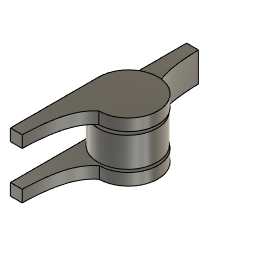
My_hinge (Autodesk Fusion 360 design; units mm, degrees)
Autodesk Fusion 360 part; units mm, degrees
sketch "Sketch1" plane through (0, 0, 0) normal (0, 0, 1) x (1, 0, 0)
  line L0 (-3, 15) -> (-5, 15)
  line L1 (-5, 15) -> (-5, 0)
  line L2 (-3, -30) -> (-3, -30)
  line L3 (-3, -30) -> (-5, -30)
  line L4 (-5, -30) -> (-5, -15)
  spline S0 degree 5 poles (-3, 15) (-2.9929, 14.7028) (-2.9742, 14.1164) (-2.9328, 13.2606) (-2.8507, 12.1683) (-2.6998, 10.89) (-2.4955, 9.708) (-2.2318, 8.6329) (-1.9035, 7.6743) (-1.5088, 6.8353) (-1.0507, 6.1105) (-0.6369, 5.6161) (-0.3014, 5.2906) (-0.0668, 5.0934) (0.0533, 4.9997) knots 0 0 0 0 0 0 0.1 0.2 0.3 0.4 0.5 0.6 0.7 0.8 0.9 1 1 1 1 1 1
  spline S1 degree 5 poles (-3, -30) (-2.9942, -29.702) (-2.978, -29.114) (-2.9397, -28.2561) (-2.8602, -27.1614) (-2.7099, -25.8808) (-2.5033, -24.6975) (-2.2343, -23.6219) (-1.8972, -22.6638) (-1.4903, -21.8261) (-1.0169, -21.1033) (-0.5884, -20.6109) (-0.2406, -20.2872) (0.0028, -20.0913) (0.1274, -19.9984) knots 0 0 0 0 0 0 0.1 0.2 0.3 0.4 0.5 0.6 0.7 0.8 0.9 1 1 1 1 1 1
  arc A0 (-5, 0) -> (0.0533, 4.9997) centre (0, 0) ccw
  arc A1 (0.1274, -19.9984) -> (-5, -15) centre (0, -15) ccw
  circle A2 centre (0, 0) radius 2.5
  circle A3 centre (0, -15) radius 2.25
  point P0 (-2, 8)
  point P1 (-2, -23)
  dimension "d1" = 10
  dimension "d2" = 10
  dimension "d3" = 5
  dimension "d4" = 4.5
  constraint coincident A0.centre A2.centre
  constraint tangent L1 A0
  constraint vertical L2
  constraint perpendicular L2 L3
  constraint tangent L4 A1
  constraint coincident S1 L2.start
  measures "d1" diameter of A0
  measures "d2" diameter of A1
  measures "d3" diameter of A2
  measures "d4" diameter of A3
extrude "Extrude1" add sketch "Sketch1" along normal blind 5 contours L0 L1 S0 A0 makes body 1
sketch "Sketch2" plane through (0, 0, 0) normal (0, 0, 1) x (1, 0, 0)
  line L0 (-5, -30) -> (-5, -15)
  line L1 (-5, -30) -> (-3, -30)
  spline S0 degree 5 poles (-3, -30) (-2.9918, -29.7034) (-2.9712, -29.1182) (-2.9275, -28.2641) (-2.8434, -27.1736) (-2.6919, -25.8969) (-2.4892, -24.7158) (-2.2296, -23.641) (-1.908, -22.682) (-1.5227, -21.842) (-1.0765, -21.1155) (-0.6739, -20.6194) (-0.3479, -20.2925) (-0.1199, -20.0942) (-0.0033, -20) knots 0 0 0 0 0 0 0.1 0.2 0.3 0.4 0.5 0.6 0.7 0.8 0.9 1 1 1 1 1 1
  arc A0 (-0.0033, -20) -> (-5, -15) centre (0, -15) ccw
  point P0 (-2, -23)
  dimension "d7" = 10
  dimension "d8" = 2
  constraint tangent L0 A0
  constraint perpendicular L0 L1
  measures "d7" diameter of A0
  measures "d8" distance of L0.start L1.end
extrude "Extrude2" add sketch "Sketch2" along normal blind 2 separate body makes body 2
sketch "Sketch3" plane through (0, 0, 0) normal (0, 0, 1) x (1, 0, 0)
  line L0 (0, 10) -> (0, 25)
  line L1 (0, 10) -> (2, 10)
  spline S0 degree 5 poles (2, 10) (2.0091, 10.296) (2.0314, 10.8803) (2.0772, 11.733) (2.1631, 12.822) (2.315, 14.0973) (2.5163, 15.2775) (2.7724, 16.3521) (3.0882, 17.3115) (3.4655, 18.1525) (3.9015, 18.8805) (4.2942, 19.3781) (4.6121, 19.7063) (4.8342, 19.9056) (4.9478, 20.0003) knots 0 0 0 0 0 0 0.1 0.2 0.3 0.4 0.5 0.6 0.7 0.8 0.9 1 1 1 1 1 1
  arc A0 (4.9478, 20.0003) -> (0, 25) centre (5, 25) ccw
  circle A1 centre (0, -15) radius 2.25
  point P0 (3, 17)
  dimension "d11" = 10
  dimension "d12" = 2
  dimension "d13" = 4.5
  constraint tangent L0 A0
  constraint perpendicular L0 L1
  measures "d11" diameter of A0
  measures "d12" distance of L0.start L1.end
  measures "d13" diameter of A1
extrude "Extrude3" add sketch "Sketch3" against normal blind 9 contours A1 bodies 2
extrude "Extrude4" cut 1 faces at (0.6157, -14.0527, -9) along direction (0, 0, 1) blind 3 on bodies 2 bodies 2
sketch "Sketch4" plane through (0, 0, -6) normal (0, 0, -1) x (1, 0, 0)
  circle A0 centre (0, 15) radius 2.25
  line L0 (-3, 30) -> (-5, 30)
  line L1 (-5, 30) -> (-5, 15)
  spline S0 degree 5 poles (-3, 30) (-2.9933, 29.7025) (-2.9754, 29.1156) (-2.9351, 28.2591) (-2.8539, 27.166) (-2.7032, 25.887) (-2.4981, 24.7045) (-2.2326, 23.6293) (-1.9014, 22.6709) (-1.5027, 21.8323) (-1.0396, 21.1082) (-0.6209, 20.6145) (-0.2813, 20.2896) (-0.0437, 20.0928) (0.0779, 19.9994) knots 0 0 0 0 0 0 0.1 0.2 0.3 0.4 0.5 0.6 0.7 0.8 0.9 1 1 1 1 1 1
  arc A1 (-5, 15) -> (0.0779, 19.9994) centre (0, 15) ccw
  point P0 (-2, 23)
  dimension "d18" = 10
  constraint concentric A0 A1
  constraint tangent L1 A1
  measures "d18" diameter of A1
extrude "Extrude5" add sketch "Sketch4" along normal blind 2 separate body makes body 3
extrude "Extrude6" add 1 faces at (0.6157, -14.0527, -6) along direction (0, 0, -1) blind 2 on bodies 2 bodies 2 3
move_body "Move1" bodies 1 to x (1, 0, 0) y (0, 1, 0) z (0, 0, 1) at (7.9171, -16.1654, -6.25)
move_body "Move2" bodies 1 to x (1, 0, 0) y (0, 1, 0) z (0, 0, 1) at (-7.9938, -2.8896, 0.7)
move_body "Move3" bodies 1 to x (1, 0, 0) y (0, 1, 0) z (0, 0, 1) at (0, 4, 0)
